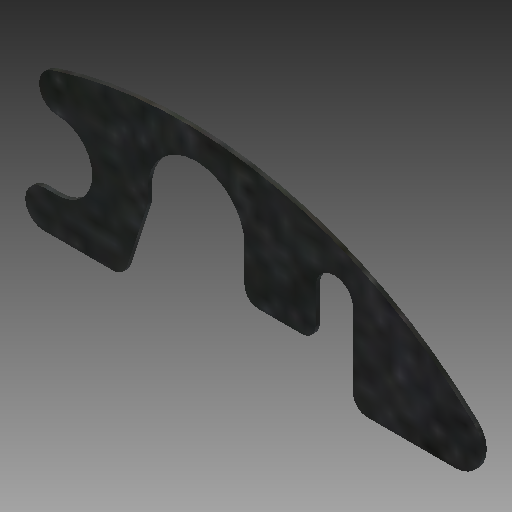
# Autodesk Inventor part: 308-15
Saved by Autodesk Inventor 2019 (Build 230136000, 136)
## iProperties
Company: Autodesk Inc.
Created: 2012-01-24
Part Number: 308-15
Material: Steel
Document SubType Name: Modeling
Designer: Autodesk Inc.
Mass: 0.455007 g
Surface Area: 4.18377 cm^2
Volume: 0.0579626 cm^3
Density: 7.85 g/cm^3
Appearance: Plate
Author: Inventor
Autodesk Inventor part; units mm, degrees
ref_plane "YZ Plane" through (0, 0, 0) normal (1, 0, 0) x (0, 1, 0)
ref_plane "XZ Plane" through (0, 0, 0) normal (0, 1, 0) x (-1, 0, 0)
ref_plane "XY Plane" through (0, 0, 0) normal (0, 0, 1) x (1, 0, 0)
sketch "Sketch1" plane through (0, 0, 0) normal (0, 0, 1) x (1, 0, 0)
  circle A0 centre (0, 0) radius 3.5
  circle A1 centre (10, 0) radius 1.35
  circle A2 centre (18.7217, -4.35) radius 2
  line L0 (-3.5, 0) -> (-3.5, -1)
  line L1 (-3.5, -1) -> (-5.2383, -6.35)
  line L2 (-5.2383, -6.35) -> (-11, -6.35)
  line L3 (3.5, 0) -> (3.5, -3.5)
  line L4 (3.5, -3.5) -> (8.65, -3.5)
  line L5 (8.65, -3.5) -> (8.65, 0)
  arc A3 (20.1001, -2.9009) -> (-10.4205, 3.9828) centre (-0.9208, -25) ccw
  circle A4 centre (-10, 2.7) radius 1.35
  circle A5 centre (-11, -5) radius 1.35
  line L6 (18.7217, -6.35) -> (11.35, -6.35)
  line L7 (11.35, -6.35) -> (11.35, 0)
  line L8 (-11, -3.65) -> (-10, -3.65)
  arc A6 (-10, -3.65) -> (-10, 1.35) centre (-10, -1.15) ccw
  line L9 (-10, 1.35) -> (-10, 1.35)
  dimension "d0" = 3.5
  dimension "d1" = 1.35
  dimension "d2" = 10
  dimension "d5" = 1
  dimension "d6" = 30.5
  dimension "d10" = 20
  dimension "d15" = 21.5
  dimension "d16" = 18
  dimension "d18" = 2
  dimension "d20" = 10
  dimension "d21" = 11
  dimension "d22" = 2.5
  constraints: 20 end point, 14 point on circle, 13 tangent, 7 centre point, 3 parallel, 3 vertical, 2 collinear, 2 equal radius, 2 horizontal, 1 coincident, 1 horizontal alignment, 1 vertical alignment
  measures "d0" radius of A0
  measures "d1" radius of A1
  measures "d2" distance of A1.centre A0.centre
  measures "d5" distance of L0.start L0.end
  measures "d6" radius of A3
  measures "d10" vertical distance of A5.centre A3.centre
  measures "d15" distance from line of L4 A3.centre
  measures "d16" angle of L3 L1
  measures "d18" radius of A2
  measures "d20" horizontal distance of point (0, 0) A4.centre
  measures "d21" horizontal distance of point (0, 0) A5.centre
  measures "d22" radius of A6
extrude "Extrusion1" add sketch "Sketch1" along normal blind 0.3 contours A0 L0 L1 L2 A5 L8 A6 A4 A3 A2 L6 L7 A1 L5 L4 L3 | A5 | A2 | A4
fillet "Fillet1" radius 1 5 edges at (-5.2383, -6.35, 0.15) (-3.5, -1, 0.15) (3.5, -3.5, 0.15) (8.65, -3.5, 0.15) (11.35, -6.35, 0.15)
body "Solid1"
